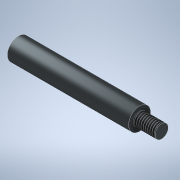
# Autodesk Inventor part: Bolzen
Saved by Autodesk Inventor 2021 (Build 250183000, 183)
## iProperties
Created: 2022-04-22
Part Number: Bolzen
Material: Eisen, Grau
Document SubType Name: Modeling
Designer: Timo
Density: 7.15 g/cm^3
Appearance: Eisen - Grau
Mass: 33.0871 g
Surface Area: 20.9858 cm^2
Volume: 4.62757 cm^3
Author: Timo
Autodesk Inventor part; units mm, degrees
ref_plane "YZ Plane" through (0, 0, 0) normal (1, 0, 0) x (0, 1, 0)
ref_plane "XZ Plane" through (0, 0, 0) normal (0, 1, 0) x (-1, 0, 0)
ref_plane "XY Plane" through (0, 0, 0) normal (0, 0, 1) x (1, 0, 0)
sketch "Skizze1" plane through (0, 0, 0) normal (0, 0, 1) x (1, 0, 0)
  line L0 (10, 0) -> (-48, 0)
  line L1 (-55, 5) -> (0, 5)
  line L2 (0, 5) -> (0, 3)
  line L3 (0, 3) -> (10, 3)
  line L4 (10, 3) -> (10, 0)
  line L5 (-55, 5) -> (-55, 2)
  line L6 (-55, 2) -> (-48, 2)
  line L7 (-48, 2) -> (-48, 0)
  point P0 (0, 0)
  point P1 (0, 4)
  dimension "d0" = 10
  dimension "d2" = 10
  dimension "d3" = 6
  dimension "d8" = 55
  dimension "d9" = 4
  dimension "d12" = 7
  constraints: 16 end point, 3 perpendicular, 2 horizontal, 2 vertical, 1 midpoint, 1 point on line, 1 vertical alignment
  measures "d0" diameter of L1 L0
  measures "d2" distance of L2.end L3.end
  measures "d3" diameter of L3 L0
  measures "d8" distance of L1.start L1.end
  measures "d9" diameter of L6 L0
  measures "d12" distance between parallel lines of L7 L5
revolve "Umdrehung1" add sketch "Skizze1" angle 360 about axis through (10, 0, 0) along (-1, 0, 0)
thread "Gewinde2" size "M6x1" class "6g" standard "ANSI Metric M Profile" length 28
thread "Gewinde3" size "M4x0.7" class "6H" standard "ANSI Metric M Profile" full length
